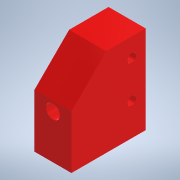
# Autodesk Inventor part: innerbracket
Saved by Autodesk Inventor 2020.1 (Build 241239000, 239)
## iProperties
Created: 2019-12-09
Part Number: innerbracket
Material: ABS Plastic
Document SubType Name: Modeling
Designer: tbloo
Density: 1.06 g/cm^3
Appearance: Smooth - Red
Author: tbloo
Autodesk Inventor part; units mm, degrees
ref_plane "YZ Plane" through (0, 0, 0) normal (1, 0, 0) x (0, 1, 0)
ref_plane "XZ Plane" through (0, 0, 0) normal (0, 1, 0) x (-1, 0, 0)
ref_plane "XY Plane" through (0, 0, 0) normal (0, 0, 1) x (1, 0, 0)
sketch "Sketch1" plane through (0, 0, 0) normal (0, 1, 0) x (-1, 0, 0)
  line L0 (0, 0) -> (16, 0)
  line L1 (16, 0) -> (16, -32)
  line L2 (16, -32) -> (0, -32)
  line L3 (0, -32) -> (0, 0)
  dimension "d0" = 16
  dimension "d1" = 32
  constraints: 8 end point, 2 parallel, 1 horizontal, 1 perpendicular
  measures "d0" distance of L1.end L2.end
  measures "d1" distance of L0.end L1.end
extrude "Extrusion1" add sketch "Sketch1" along normal blind 38
sketch "Sketch2" plane through (-16, 0, -32) normal (-1, 0, 0) x (0, 0, 1)
  circle A0 centre (6, 14) radius 1.3525
  circle A1 centre (6, 30) radius 1.3525
  point P0 (32, 0)
  constraints: 2 centre point, 4 other
hole "Hole1" at (-16, 14, -26) at (-16, 30, -26) direction (1, 0, 0) diameter 3.7 end through all counterbore diameter 6 counterbore depth 10
sketch "Sketch3" plane through (0, 0, 0) normal (0, -1, 0) x (1, 0, 0)
  circle A0 centre (-8, -25) radius 1.85
  circle A1 centre (-8, -9) radius 1.85
  point P0 (0, 0)
  constraints: 2 centre point, 4 other
hole "Hole2" at (-8, 0, -25) at (-8, 0, -9) direction (0, 1, 0) diameter 3.7 depth 8
chamfer "Chamfer1" distance 15 angle 45 1 edges at (-8, 38, 0)
sketch "Sketch4" plane through (0, 0, -32) normal (0, 0, -1) x (-1, 0, 0)
  line L0 (0, 0) -> (16, 0)
  line L1 (16, 0) -> (16, 38)
  line L2 (0, 38) -> (16, 38)
  line L3 (0, 0) -> (0, 38)
  point P0 (8, 19)
  constraints: 8 end point
hole "Hole3" at (-8, 19, -32) direction (0, 0, 1) diameter 3.7 end through all
sketch "Sketch6" plane through (-16, 0, 0) normal (0, 0, 1) x (1, 0, 0)
  circle A0 centre (8, 19) radius 1.85
  point P0 (16, 0)
  constraints: 1 centre point
hole "Hole5" at (-8, 19, 0) direction (0, 0, -1) diameter 6 depth 10
body "Solid1"
